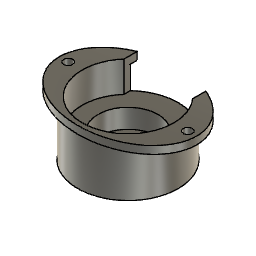
speaker_holder v1 (Autodesk Fusion 360 design; units mm, degrees)
Autodesk Fusion 360 part; units mm, degrees
sketch "Sketch1" plane through (0, 0, 0) normal (0, 0, 1) x (1, 0, 0)
  circle A0 centre (0, 0) radius 19.75
  dimension "d1" = 39.5
  constraint coincident A0.centre origin
  measures "d1" diameter of A0
extrude "Extrude1" add sketch "Sketch1" along normal blind 2
sketch "Sketch2" plane through (0, 0, 2) normal (0, 0, 1) x (-1, 0, 0)
  circle A0 centre (0, 0) radius 19.75
  circle A1 centre (0, 0) radius 11.75
  circle A2 centre (0, 0) radius 19.75
  dimension "d4" = 23.5
  constraint coincident A0.centre A1.centre
  measures "d4" diameter of A1
extrude "Extrude2" add sketch "Sketch2" along normal blind 7.5
sketch "Sketch3" plane through (0, 0, 9.5) normal (0, 0, 1) x (-1, 0, 0)
  circle A0 centre (0, 0) radius 11.75
  circle A1 centre (0, 0) radius 19.75
  circle A2 centre (0, 0) radius 19.75
  circle A3 centre (0, 0) radius 18
  dimension "d7" = 36
  constraint coincident A0.centre A1.centre
  measures "d7" diameter of A3
extrude "Extrude3" add sketch "Sketch3" along normal blind 12 contours A1 A2
sketch "Sketch4" plane through (0, 0, 21.5) normal (0, 0, 1) x (-1, 0, 0)
  circle A0 centre (0, 0) radius 18
  circle A1 centre (0, 0) radius 19.75
  circle A2 centre (0, 0) radius 19.75
  line L0 (-27, -19.75) -> (27, -19.75)
  line L1 (27, -19.75) -> (27, 19.75)
  line L2 (27, 19.75) -> (-27, 19.75)
  line L3 (-27, 19.75) -> (-27, -19.75)
  line L4 (-27, -19.75) -> (27, 19.75) construction
  line L5 (27, -19.75) -> (-27, 19.75) construction
  line L6 (-27, 0) -> (-23.5, 0)
  line L7 (27, 0) -> (23.5, 0)
  circle A3 centre (23.5, 0) radius 1.75
  circle A4 centre (-23.5, 0) radius 1.75
  dimension "d10" = 39.5
  dimension "d11" = 54
  dimension "d12" = 3.5
  dimension "d13" = 3.5
  dimension "d14" = 3.5
  dimension "d15" = 3.5
  constraint concentric A0 A2
  constraint horizontal L0
  constraint perpendicular L0 L1
  constraint parallel L0 L2
  constraint parallel L1 L3
  constraint coincident L4 A0.centre
  constraint coincident L5 A0.centre
  constraint coincident A0.centre A1.centre
  constraint midpoint L3 L6.start
  constraint perpendicular L3 L6
  constraint midpoint L1 L7.start
  constraint perpendicular L1 L7
  constraint coincident L7.end A3.centre
  constraint coincident L6.end A4.centre
  measures "d10" distance of L0.start L2.end
  measures "d11" distance of L1.end L2.end
  measures "d12" distance of L6.start L6.end
  measures "d13" distance of L7.start L7.end
  measures "d14" diameter of A3
  measures "d15" diameter of A4
extrude "Extrude4" add sketch "Sketch4" against normal blind 3 contours A1 A2 L0 L1 L2 | A1 A2 L0 L2 L3
sketch "Sketch5" plane through (0, 0, 21.5) normal (0, 0, 1) x (-1, 0, 0)
  circle A0 centre (23.5, 0) radius 1.75
  circle A1 centre (-23.5, 0) radius 1.75
  circle A2 centre (0, 0) radius 18
  line L0 (-27, -19.75) -> (27, -19.75)
  line L1 (27, -19.75) -> (27, 19.75)
  line L2 (27, 19.75) -> (-27, 19.75)
  line L3 (-27, 19.75) -> (-27, -19.75)
  ellipse E0 centre (0, 0) end of major axis (-27, 0) minor radius 19.75
  line L4 (27, 0) -> (-27, 0) construction
  line L5 (0, 19.75) -> (0, -19.75) construction
  line L6 (27, -19.75) -> (-27, -19.75)
  line L7 (-27, -19.75) -> (-27, 19.75)
  line L8 (-27, 19.75) -> (27, 19.75)
  line L9 (27, 19.75) -> (27, -19.75)
  constraint coincident E0 L4.start
  constraint coincident E0 L4.end
  constraint coincident E0 L5.start
  constraint coincident E0 L5.end
  constraint concentric A2 E0
  constraint perpendicular L3 L4
  constraint horizontal L6
  constraint vertical L7
  constraint horizontal L8
  constraint vertical L9
  constraint coincident L2.end L3.start
  constraint coincident L0.end L1.start
extrude "Extrude5" cut sketch "Sketch5" against normal blind 10 contours L0 L3 E0 L6 L7 | L0 L1 E0 L6 L9 | L2 L3 E0 L7 L8 | L1 L2 E0 L8 L9
ref_plane "WorkPlane1" through (0, 11.75, 7.4179) normal (0, -1, 0) x (-1, 0, 0)
ref_plane "WorkPlane2" through (0, 17.75, 7.4179) normal (0, -1, 0) x (-1, 0, 0)
sketch "Sketch6" plane through (0, 17.75, 0) normal (0, -1, 0) x (-1, 0, 0)
  line L0 (0, 0) -> (0, -15.5)
  line L1 (-30, -21.5) -> (30, -21.5)
  line L2 (30, -21.5) -> (30, -9.5)
  line L3 (30, -9.5) -> (-30, -9.5)
  line L4 (-30, -9.5) -> (-30, -21.5)
  line L5 (-30, -21.5) -> (30, -9.5) construction
  line L6 (30, -21.5) -> (-30, -9.5) construction
  line L7 (30, -21.5) -> (-30, -21.5)
  line L8 (-30, -21.5) -> (-30, -35.9601)
  line L9 (-30, -35.9601) -> (30, -35.9601)
  line L10 (30, -35.9601) -> (30, -21.5)
  point P0 (0, -15.5)
  dimension "d22" = 15.5
  dimension "d23" = 12
  dimension "d24" = 60
  dimension "d25" = 60
  constraint coincident L0.start origin
  constraint vertical L0
  constraint horizontal L1
  constraint perpendicular L1 L2
  constraint parallel L1 L3
  constraint parallel L2 L4
  constraint coincident L5 P0
  constraint coincident L6 P0
  constraint coincident P0 L0.end
  constraint horizontal L7
  constraint vertical L8
  constraint horizontal L9
  constraint vertical L10
  measures "d22" distance of L0.start P0
  measures "d23" distance of L1.start L3.end
  measures "d24" distance of L2.end L3.end
  measures "d25" distance of L8.end L9.end
extrude "Extrude6" cut sketch "Sketch6" against normal blind 20
sketch "Sketch7" plane through (0, 17.75, 0) normal (0, 1, 0) x (-1, 0, 0)
  line L0 (-8.6603, 18.5) -> (-8.6603, 9.5)
  line L1 (-8.6603, 9.5) -> (-2.9896, 9.5)
  line L2 (-2.9896, 9.5) -> (-2.9896, 21.5)
  line L3 (-2.9896, 21.5) -> (-11.8393, 21.5)
  line L4 (-11.8393, 21.5) -> (-11.8393, 18.5)
  line L5 (-11.8393, 18.5) -> (-8.6603, 18.5)
  line L6 (13.5, 23.7273) -> (-13.5, 23.7273)
  line L7 (-13.5, 23.7273) -> (-13.5, -4.7273)
  line L8 (-13.5, -4.7273) -> (13.5, -4.7273)
  line L9 (13.5, -4.7273) -> (13.5, 23.7273)
  line L10 (13.5, 23.7273) -> (-13.5, -4.7273) construction
  line L11 (-13.5, 23.7273) -> (13.5, -4.7273) construction
  line L12 (0, 9.5) -> (13.5, 9.5)
  line L13 (0, 9.5) -> (-13.5, 9.5)
  point P0 (0, 9.5)
  dimension "d28" = 27
  constraint horizontal L6
  constraint perpendicular L6 L7
  constraint parallel L6 L8
  constraint parallel L7 L9
  constraint coincident L10 P0
  constraint coincident L11 P0
  constraint coincident P0 L12.start
  constraint midpoint L9 L12.end
  constraint perpendicular L9 L12
  constraint midpoint L7 L13.end
  measures "d28" distance of L6.start L6.end
extrude "Extrude7" cut sketch "Sketch7" against normal blind 20 contours L0 L1 L2 L3 L4 L5 L13 | L0 L2 L3 L4 L5 L6 L7 L9 L12 L13
